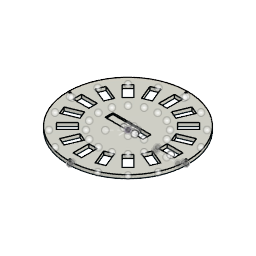
main (Autodesk Fusion 360 design; units mm, degrees)
Autodesk Fusion 360 part; units mm, degrees
sketch "Sketch1" plane through (0, 0, 0) normal (0, 0, 1) x (1, 0, 0)
  circle A0 centre (0, 0) radius 85
  line L0 (0, -85) -> (-7, -85) construction
  line L1 (0, -85) -> (7, -85) construction
  line L2 (-7, -85) -> (-7, -82) construction
  line L3 (7, -85) -> (7, -82) construction
  line L4 (7, -77) -> (5.9, -77) construction
  line L5 (7, -44.8) -> (5.9, -44.8) construction
  line L6 (-7, -44.8) -> (-5.9, -44.8) construction
  line L7 (-5.9, -44.8) -> (5.9, -44.8)
  line L8 (5.9, -44.8) -> (5.9, -77)
  line L9 (5.9, -77) -> (-5.9, -77)
  line L10 (-5.9, -77) -> (-5.9, -44.8)
  line L11 (0, -39.8) -> (0, -44.8) construction
  line L12 (11.6933, -43.6476) -> (22.5951, -39.132)
  line L13 (24.0157, -73.3966) -> (11.6933, -43.6476)
  line L14 (22.5951, -39.132) -> (34.9175, -68.8809)
  line L15 (34.9175, -68.8809) -> (24.0157, -73.3966)
  line L16 (27.5065, -35.8503) -> (35.8503, -27.5065)
  line L17 (50.2753, -58.6192) -> (27.5065, -35.8503)
  line L18 (35.8503, -27.5065) -> (58.6192, -50.2753)
  line L19 (58.6192, -50.2753) -> (50.2753, -58.6192)
  line L20 (39.132, -22.5951) -> (43.6476, -11.6933)
  line L21 (68.8809, -34.9175) -> (39.132, -22.5951)
  line L22 (43.6476, -11.6933) -> (73.3966, -24.0157)
  line L23 (73.3966, -24.0157) -> (68.8809, -34.9175)
  line L24 (44.8, -5.9) -> (44.8, 5.9)
  line L25 (77, -5.9) -> (44.8, -5.9)
  line L26 (44.8, 5.9) -> (77, 5.9)
  line L27 (77, 5.9) -> (77, -5.9)
  line L28 (43.6476, 11.6933) -> (39.132, 22.5951)
  line L29 (73.3966, 24.0157) -> (43.6476, 11.6933)
  line L30 (39.132, 22.5951) -> (68.8809, 34.9175)
  line L31 (68.8809, 34.9175) -> (73.3966, 24.0157)
  line L32 (35.8503, 27.5065) -> (27.5065, 35.8503)
  line L33 (58.6192, 50.2753) -> (35.8503, 27.5065)
  line L34 (27.5065, 35.8503) -> (50.2753, 58.6192)
  line L35 (50.2753, 58.6192) -> (58.6192, 50.2753)
  line L36 (22.5951, 39.132) -> (11.6933, 43.6476)
  line L37 (34.9175, 68.8809) -> (22.5951, 39.132)
  line L38 (11.6933, 43.6476) -> (24.0157, 73.3966)
  line L39 (24.0157, 73.3966) -> (34.9175, 68.8809)
  line L40 (5.9, 44.8) -> (-5.9, 44.8)
  line L41 (5.9, 77) -> (5.9, 44.8)
  line L42 (-5.9, 44.8) -> (-5.9, 77)
  line L43 (-5.9, 77) -> (5.9, 77)
  line L44 (-11.6933, 43.6476) -> (-22.5951, 39.132)
  line L45 (-24.0157, 73.3966) -> (-11.6933, 43.6476)
  line L46 (-22.5951, 39.132) -> (-34.9175, 68.8809)
  line L47 (-34.9175, 68.8809) -> (-24.0157, 73.3966)
  line L48 (-27.5065, 35.8503) -> (-35.8503, 27.5065)
  line L49 (-50.2753, 58.6192) -> (-27.5065, 35.8503)
  line L50 (-35.8503, 27.5065) -> (-58.6192, 50.2753)
  line L51 (-58.6192, 50.2753) -> (-50.2753, 58.6192)
  line L52 (-39.132, 22.5951) -> (-43.6476, 11.6933)
  line L53 (-68.8809, 34.9175) -> (-39.132, 22.5951)
  line L54 (-43.6476, 11.6933) -> (-73.3966, 24.0157)
  line L55 (-73.3966, 24.0157) -> (-68.8809, 34.9175)
  line L56 (-44.8, 5.9) -> (-44.8, -5.9)
  line L57 (-77, 5.9) -> (-44.8, 5.9)
  line L58 (-44.8, -5.9) -> (-77, -5.9)
  line L59 (-77, -5.9) -> (-77, 5.9)
  line L60 (-43.6476, -11.6933) -> (-39.132, -22.5951)
  line L61 (-73.3966, -24.0157) -> (-43.6476, -11.6933)
  line L62 (-39.132, -22.5951) -> (-68.8809, -34.9175)
  line L63 (-68.8809, -34.9175) -> (-73.3966, -24.0157)
  line L64 (-35.8503, -27.5065) -> (-27.5065, -35.8503)
  line L65 (-58.6192, -50.2753) -> (-35.8503, -27.5065)
  line L66 (-27.5065, -35.8503) -> (-50.2753, -58.6192)
  line L67 (-50.2753, -58.6192) -> (-58.6192, -50.2753)
  line L68 (-22.5951, -39.132) -> (-11.6933, -43.6476)
  line L69 (-34.9175, -68.8809) -> (-22.5951, -39.132)
  line L70 (-11.6933, -43.6476) -> (-24.0157, -73.3966)
  line L71 (-24.0157, -73.3966) -> (-34.9175, -68.8809)
  dimension "d1" = 170
  dimension "d2" = 7
  dimension "d3" = 7
  dimension "d4" = 3
  dimension "d5" = 3
  dimension "d7" = 5
  dimension "d8" = 1.1
  dimension "d10" = 1.1
  dimension "d11" = 1.1
  dimension "d15" = 360
  constraint coincident A0.centre origin
  constraint coincident A0 L0.start
  constraint horizontal L0
  constraint parallel L0 L1
  constraint perpendicular L0 L2
  constraint perpendicular L1 L3
  constraint perpendicular L7 L8
  constraint parallel L7 L9
  constraint parallel L8 L10
  constraint parallel L5 L7
  constraint midpoint L7 L11.end
  measures "d1" diameter of A0
  measures "d2" distance of L0.start L0.end
  measures "d3" distance of L0.start L1.end
  measures "d4" distance of L0.end L2.end
  measures "d5" distance of L1.end L3.end
  measures "d7" distance of L3.end L4.start
  measures "d8" distance of L4.start L4.end
  measures "d10" distance of L5.start L5.end
  measures "d11" distance of L6.start L6.end
extrude "Extrude1" add sketch "Sketch1" along normal blind 5
sketch "Sketch2" plane through (0, 0, 5) normal (0, 0, 1) x (-1, 0, 0)
  line L0 (-27.5065, -35.8503) -> (-50.2753, -58.6192)
  line L1 (-50.2753, -58.6192) -> (-58.6192, -50.2753)
  line L2 (-58.6192, -50.2753) -> (-35.8503, -27.5065)
  line L3 (-35.8503, -27.5065) -> (-27.5065, -35.8503)
  line L4 (5.9, -44.8) -> (5.9, -77)
  line L5 (5.9, -77) -> (-5.9, -77)
  line L6 (-5.9, -77) -> (-5.9, -44.8)
  line L7 (-5.9, -44.8) -> (5.9, -44.8)
  line L8 (-35.8503, 27.5065) -> (-58.6192, 50.2753)
  line L9 (-58.6192, 50.2753) -> (-50.2753, 58.6192)
  line L10 (-50.2753, 58.6192) -> (-27.5065, 35.8503)
  line L11 (-27.5065, 35.8503) -> (-35.8503, 27.5065)
  line L12 (35.8503, -27.5065) -> (58.6192, -50.2753)
  line L13 (58.6192, -50.2753) -> (50.2753, -58.6192)
  line L14 (50.2753, -58.6192) -> (27.5065, -35.8503)
  line L15 (27.5065, -35.8503) -> (35.8503, -27.5065)
  circle A0 centre (0, 0) radius 85
  line L16 (-5.9, 77) -> (5.9, 77)
  line L17 (5.9, 77) -> (5.9, 44.8)
  line L18 (5.9, 44.8) -> (-5.9, 44.8)
  line L19 (-5.9, 44.8) -> (-5.9, 77)
  line L20 (-39.132, -22.5951) -> (-68.8809, -34.9175)
  line L21 (-68.8809, -34.9175) -> (-73.3966, -24.0157)
  line L22 (-73.3966, -24.0157) -> (-43.6476, -11.6933)
  line L23 (-43.6476, -11.6933) -> (-39.132, -22.5951)
  line L24 (22.5951, -39.132) -> (34.9175, -68.8809)
  line L25 (34.9175, -68.8809) -> (24.0157, -73.3966)
  line L26 (24.0157, -73.3966) -> (11.6933, -43.6476)
  line L27 (11.6933, -43.6476) -> (22.5951, -39.132)
  line L28 (39.132, 22.5951) -> (68.8809, 34.9175)
  line L29 (68.8809, 34.9175) -> (73.3966, 24.0157)
  line L30 (73.3966, 24.0157) -> (43.6476, 11.6933)
  line L31 (43.6476, 11.6933) -> (39.132, 22.5951)
  line L32 (-22.5951, 39.132) -> (-34.9175, 68.8809)
  line L33 (-34.9175, 68.8809) -> (-24.0157, 73.3966)
  line L34 (-24.0157, 73.3966) -> (-11.6933, 43.6476)
  line L35 (-11.6933, 43.6476) -> (-22.5951, 39.132)
  line L36 (44.8, 5.9) -> (77, 5.9)
  line L37 (77, 5.9) -> (77, -5.9)
  line L38 (77, -5.9) -> (44.8, -5.9)
  line L39 (44.8, -5.9) -> (44.8, 5.9)
  line L40 (-11.6933, -43.6476) -> (-24.0157, -73.3966)
  line L41 (-24.0157, -73.3966) -> (-34.9175, -68.8809)
  line L42 (-34.9175, -68.8809) -> (-22.5951, -39.132)
  line L43 (-22.5951, -39.132) -> (-11.6933, -43.6476)
  line L44 (-43.6476, 11.6933) -> (-73.3966, 24.0157)
  line L45 (-73.3966, 24.0157) -> (-68.8809, 34.9175)
  line L46 (-68.8809, 34.9175) -> (-39.132, 22.5951)
  line L47 (-39.132, 22.5951) -> (-43.6476, 11.6933)
  line L48 (27.5065, 35.8503) -> (50.2753, 58.6192)
  line L49 (50.2753, 58.6192) -> (58.6192, 50.2753)
  line L50 (58.6192, 50.2753) -> (35.8503, 27.5065)
  line L51 (35.8503, 27.5065) -> (27.5065, 35.8503)
  line L52 (43.6476, -11.6933) -> (73.3966, -24.0157)
  line L53 (73.3966, -24.0157) -> (68.8809, -34.9175)
  line L54 (68.8809, -34.9175) -> (39.132, -22.5951)
  line L55 (39.132, -22.5951) -> (43.6476, -11.6933)
  line L56 (-44.8, -5.9) -> (-77, -5.9)
  line L57 (-77, -5.9) -> (-77, 5.9)
  line L58 (-77, 5.9) -> (-44.8, 5.9)
  line L59 (-44.8, 5.9) -> (-44.8, -5.9)
  line L60 (11.6933, 43.6476) -> (24.0157, 73.3966)
  line L61 (24.0157, 73.3966) -> (34.9175, 68.8809)
  line L62 (34.9175, 68.8809) -> (22.5951, 39.132)
  line L63 (22.5951, 39.132) -> (11.6933, 43.6476)
  line L64 (0, 0) -> (0, 5.5) construction
  line L65 (0, 5.5) -> (27, 5.5) construction
  line L66 (27, 5.5) -> (27, -5.5) construction
  line L67 (27, -5.5) -> (-27, -5.5) construction
  line L68 (27, 5.5) -> (27, -5.5)
  line L69 (27, -5.5) -> (-27, -5.5)
  line L70 (-27, -5.5) -> (-27, 5.5)
  line L71 (-27, 5.5) -> (27, 5.5)
  dimension "d22" = 5.5
  dimension "d23" = 27
  dimension "d24" = 11
  dimension "d25" = 54
  constraint coincident A0.centre L64.start
  constraint vertical L64
  constraint perpendicular L64 L65
  constraint perpendicular L65 L66
  constraint perpendicular L66 L67
  constraint perpendicular L68 L69
  constraint parallel L68 L70
  constraint parallel L69 L71
  measures "d22" distance of A0.centre L64.end
  measures "d23" distance of L64.end L65.end
  measures "d24" distance of L65.end L66.end
  measures "d25" distance of L66.end L67.end
extrude "Extrude2" cut sketch "Sketch2" against normal blind 2 contours L68 L69 L70 L71
sketch "Sketch3" plane through (0, 0, 3) normal (0, 0, 1) x (-1, 0, 0)
  line L0 (-27, 5.5) -> (-27, -5.5)
  line L1 (-27, -5.5) -> (27, -5.5)
  line L2 (27, -5.5) -> (27, 5.5)
  line L3 (27, 5.5) -> (-27, 5.5)
  line L4 (-27, -5.5) -> (-12.1144, -5.5)
  line L5 (-12.1144, -5.5) -> (-12.1144, 5.5)
  line L6 (-12.1144, 5.5) -> (-27, 5.5)
  line L7 (-27, 5.5) -> (-27, -5.5)
  constraint horizontal L4
  constraint vertical L5
  constraint horizontal L6
  constraint vertical L7
  constraint coincident L3 L5.end
  constraint coincident L0.end L1.start
extrude "Extrude3" cut sketch "Sketch3" against normal blind 39 contours L0 L1 L3 L4 L5 L6 L7
sketch "Sketch4" plane through (0, 0, 0) normal (0, 0, -1) x (1, 0, 0)
  line L0 (-24.0157, 73.3966) -> (-11.6933, 43.6476)
  line L1 (-11.6933, 43.6476) -> (-22.5951, 39.132)
  line L2 (-22.5951, 39.132) -> (-34.9175, 68.8809)
  line L3 (-34.9175, 68.8809) -> (-24.0157, 73.3966)
  line L4 (77, -5.9) -> (44.8, -5.9)
  line L5 (44.8, -5.9) -> (44.8, 5.9)
  line L6 (44.8, 5.9) -> (77, 5.9)
  line L7 (77, 5.9) -> (77, -5.9)
  line L8 (-73.3966, -24.0157) -> (-43.6476, -11.6933)
  line L9 (-43.6476, -11.6933) -> (-39.132, -22.5951)
  line L10 (-39.132, -22.5951) -> (-68.8809, -34.9175)
  line L11 (-68.8809, -34.9175) -> (-73.3966, -24.0157)
  line L12 (-50.2753, 58.6192) -> (-27.5065, 35.8503)
  line L13 (-27.5065, 35.8503) -> (-35.8503, 27.5065)
  line L14 (-35.8503, 27.5065) -> (-58.6192, 50.2753)
  line L15 (-58.6192, 50.2753) -> (-50.2753, 58.6192)
  line L16 (73.3966, 24.0157) -> (43.6476, 11.6933)
  line L17 (43.6476, 11.6933) -> (39.132, 22.5951)
  line L18 (39.132, 22.5951) -> (68.8809, 34.9175)
  line L19 (68.8809, 34.9175) -> (73.3966, 24.0157)
  line L20 (24.0157, -73.3966) -> (11.6933, -43.6476)
  line L21 (11.6933, -43.6476) -> (22.5951, -39.132)
  line L22 (22.5951, -39.132) -> (34.9175, -68.8809)
  line L23 (34.9175, -68.8809) -> (24.0157, -73.3966)
  line L24 (-77, 5.9) -> (-44.8, 5.9)
  line L25 (-44.8, 5.9) -> (-44.8, -5.9)
  line L26 (-44.8, -5.9) -> (-77, -5.9)
  line L27 (-77, -5.9) -> (-77, 5.9)
  line L28 (34.9175, 68.8809) -> (22.5951, 39.132)
  line L29 (22.5951, 39.132) -> (11.6933, 43.6476)
  line L30 (11.6933, 43.6476) -> (24.0157, 73.3966)
  line L31 (24.0157, 73.3966) -> (34.9175, 68.8809)
  line L32 (-68.8809, 34.9175) -> (-39.132, 22.5951)
  line L33 (-39.132, 22.5951) -> (-43.6476, 11.6933)
  line L34 (-43.6476, 11.6933) -> (-73.3966, 24.0157)
  line L35 (-73.3966, 24.0157) -> (-68.8809, 34.9175)
  line L36 (-34.9175, -68.8809) -> (-22.5951, -39.132)
  line L37 (-22.5951, -39.132) -> (-11.6933, -43.6476)
  line L38 (-11.6933, -43.6476) -> (-24.0157, -73.3966)
  line L39 (-24.0157, -73.3966) -> (-34.9175, -68.8809)
  line L40 (68.8809, -34.9175) -> (39.132, -22.5951)
  line L41 (39.132, -22.5951) -> (43.6476, -11.6933)
  line L42 (43.6476, -11.6933) -> (73.3966, -24.0157)
  line L43 (73.3966, -24.0157) -> (68.8809, -34.9175)
  line L44 (-5.9, 77) -> (5.9, 77)
  line L45 (5.9, 77) -> (5.9, 44.8)
  line L46 (5.9, 44.8) -> (-5.9, 44.8)
  line L47 (-5.9, 44.8) -> (-5.9, 77)
  circle A0 centre (0, 0) radius 85
  line L48 (-58.6192, -50.2753) -> (-35.8503, -27.5065)
  line L49 (-35.8503, -27.5065) -> (-27.5065, -35.8503)
  line L50 (-27.5065, -35.8503) -> (-50.2753, -58.6192)
  line L51 (-50.2753, -58.6192) -> (-58.6192, -50.2753)
  line L52 (58.6192, 50.2753) -> (35.8503, 27.5065)
  line L53 (35.8503, 27.5065) -> (27.5065, 35.8503)
  line L54 (27.5065, 35.8503) -> (50.2753, 58.6192)
  line L55 (50.2753, 58.6192) -> (58.6192, 50.2753)
  line L56 (-5.9, -77) -> (-5.9, -44.8)
  line L57 (-5.9, -44.8) -> (5.9, -44.8)
  line L58 (5.9, -44.8) -> (5.9, -77)
  line L59 (5.9, -77) -> (-5.9, -77)
  line L60 (50.2753, -58.6192) -> (27.5065, -35.8503)
  line L61 (27.5065, -35.8503) -> (35.8503, -27.5065)
  line L62 (35.8503, -27.5065) -> (58.6192, -50.2753)
  line L63 (58.6192, -50.2753) -> (50.2753, -58.6192)
  line L64 (27, -5.5) -> (12.1144, -5.5)
  line L65 (12.1144, -5.5) -> (12.1144, 5.5)
  line L66 (12.1144, 5.5) -> (27, 5.5)
  line L67 (27, 5.5) -> (27, -5.5)
  line L68 (44.8, 0) -> (42.3, 0) construction
  line L69 (44.8, 5.9) -> (77, 5.9) construction
  line L70 (60.9, 5.9) -> (60.9, 0.1412) construction
  circle A1 centre (42.3, 0) radius 0.75
  circle A2 centre (79.5, 0) radius 0.75
  line L71 (60.9, 5.9) -> (60.9, 0.1412) construction
  circle A3 centre (73.4484, 30.4233) radius 0.75
  circle A4 centre (39.0801, 16.1875) radius 0.75
  circle A5 centre (56.215, 56.215) radius 0.75
  circle A6 centre (29.9106, 29.9106) radius 0.75
  circle A7 centre (30.4233, 73.4484) radius 0.75
  circle A8 centre (16.1875, 39.0801) radius 0.75
  circle A9 centre (0, 79.5) radius 0.75
  circle A10 centre (0, 42.3) radius 0.75
  circle A11 centre (-30.4233, 73.4484) radius 0.75
  circle A12 centre (-16.1875, 39.0801) radius 0.75
  circle A13 centre (-56.215, 56.215) radius 0.75
  circle A14 centre (-29.9106, 29.9106) radius 0.75
  circle A15 centre (-73.4484, 30.4233) radius 0.75
  circle A16 centre (-39.0801, 16.1875) radius 0.75
  circle A17 centre (-79.5, 0) radius 0.75
  circle A18 centre (-42.3, 0) radius 0.75
  circle A19 centre (-73.4484, -30.4233) radius 0.75
  circle A20 centre (-39.0801, -16.1875) radius 0.75
  circle A21 centre (-56.215, -56.215) radius 0.75
  circle A22 centre (-29.9106, -29.9106) radius 0.75
  circle A23 centre (-30.4233, -73.4484) radius 0.75
  circle A24 centre (-16.1875, -39.0801) radius 0.75
  circle A25 centre (0, -79.5) radius 0.75
  circle A26 centre (0, -42.3) radius 0.75
  circle A27 centre (30.4233, -73.4484) radius 0.75
  circle A28 centre (16.1875, -39.0801) radius 0.75
  circle A29 centre (56.215, -56.215) radius 0.75
  circle A30 centre (29.9106, -29.9106) radius 0.75
  circle A31 centre (73.4484, -30.4233) radius 0.75
  circle A32 centre (39.0801, -16.1875) radius 0.75
  line L72 (0, 79.5) -> (0, 82.5) construction
  circle A33 centre (0, 82.5) radius 1.55
  line L73 (0, 0) -> (0, 12.2218) construction
  line L74 (0, 12.2218) -> (0, 0) construction
  line L75 (0, 0) -> (-5.8676, 0) construction
  line L76 (0, 0) -> (6.7946, 0) construction
  circle A34 centre (0, -82.5) radius 1.55
  line L77 (79.5, 0) -> (82.5, 0) construction
  circle A35 centre (82.5, 0) radius 1.55
  line L78 (0, 0) -> (0, -8.2494) construction
  circle A36 centre (-82.5, 0) radius 1.55
  line L79 (0, 0) -> (-15.877, 16.4411) construction
  line L80 (0, 0) -> (22.8559, 0) construction
  line L81 (0, 0) -> (7.0711, -7.0711) construction
  line L82 (0, 0) -> (10, 0) construction
  line L83 (0, 0) -> (7.0711, 7.0711) construction
  line L84 (0, 0) -> (10, 0) construction
  line L85 (0, 0) -> (-6.6532, -6.6532) construction
  line L86 (0, 0) -> (9.4097, 0) construction
  dimension "d30" = 2.5
  dimension "d31" = 1.5
  dimension "d33" = 360
  dimension "d36" = 3
  dimension "d37" = 3.1
  dimension "d38" = 3
  dimension "d39" = 3.1
  dimension "d40" = 134
  dimension "d41" = 45
  dimension "d42" = 10
  dimension "d43" = 10
  dimension "d44" = 45
  dimension "d45" = 135
  constraint midpoint L5 L68.start
  constraint perpendicular L5 L68
  constraint coincident L5.end L6.start
  constraint coincident L6.end L7.start
  constraint midpoint L69 L70.start
  constraint perpendicular L6 L70
  constraint coincident L68.end A1.centre
  constraint symmetric L71.start L70 L70.start
  constraint symmetric L71.end L70 L70.end
  constraint symmetric L70 A1 A2
  constraint coincident A9.centre L72.start
  constraint vertical L72
  constraint coincident L72.end A33.centre
  constraint coincident A0.centre L73.start
  constraint perpendicular L66 L73
  constraint perpendicular L74 L75
  constraint perpendicular L73 L76
  constraint symmetric A33 L75 A34
  constraint coincident A2.centre L77.start
  constraint perpendicular L7 L77
  constraint coincident L77.end A35.centre
  constraint perpendicular L76 L78
  constraint symmetric A35 L78 A36
  constraint horizontal L80
  constraint horizontal L82
  constraint horizontal L84
  constraint horizontal L86
  measures "d30" distance of L68.start L68.end
  measures "d31" diameter of A1
  measures "d36" distance of A9.centre L72.end
  measures "d37" diameter of A33
  measures "d38" distance of A2.centre L77.end
  measures "d39" diameter of A35
  measures "d40" angle of L79 L80
  measures "d41" angle of L81 L82
  measures "d42" distance of A0.centre L81.end
  measures "d43" distance of A0.centre L83.end
  measures "d44" angle of L83 L84
  measures "d45" angle of L85 L86
extrude "Extrude4" cut sketch "Sketch4" against normal blind 3.5 contours A1 | A2 | A3 | A4 | A5 | A6 | A7 | A8 | A9 | A10 | A11 | A12 | A13 | A14 | A15 | A16 | A17 | A18 | A19 | A20 | A21 | A22 | A23 | A24 | A25 | A26 | A27 | A28 | A29 | A30 | A31 | A32
extrude "Extrude5" cut sketch "Sketch4" against normal blind 5 contours A33 | A34 | A35 | A36
thread "Thread1" "ISO Metric profile 3.0 M3x0.5 M3x0.5 6H" major diameter 3.086 minor diameter 2.529 pitch 0.5 angle 60 resizes the face on face at (-83.5823, -1.1096, 3.3333)
thread "Thread2" "ISO Metric profile 3.0 M3x0.5 M3x0.5 6H" major diameter 3.086 minor diameter 2.529 pitch 0.5 angle 60 resizes the face on face at (1.5481, -82.4227, 3.3333)
thread "Thread3" "ISO Metric profile 3.0 M3x0.5 M3x0.5 6H" major diameter 3.086 minor diameter 2.529 pitch 0.5 angle 60 resizes the face on face at (81.4177, -1.1096, 3.3333)
thread "Thread4" "ISO Metric profile 3.0 M3x0.5 M3x0.5 6H" major diameter 3.086 minor diameter 2.529 pitch 0.5 angle 60 resizes the face on face at (1.5481, 82.5773, 3.3333)
extrude "Extrude6" add 1 faces at (1.9667, -77, 1.6667) along direction (0, 1, 0) blind 5
extrude "Extrude7" add 1 faces at (-27.6497, -71.8913, 1.6667) along direction (0.382683, 0.92388, 0) blind 5
extrude "Extrude8" add 1 faces at (-53.0566, -55.8379, 1.6667) along direction (0.707107, 0.707107, 0) blind 5
extrude "Extrude9" add 1 faces at (-70.3861, -31.2836, 1.6667) along direction (0.92388, 0.382683, 0) blind 5
extrude "Extrude10" add 1 faces at (31.2836, -70.3861, 1.6667) along direction (-0.382683, 0.92388, 0) blind 5
extrude "Extrude11" add 1 faces at (55.8379, -53.0566, 1.6667) along direction (-0.707107, 0.707107, 0) blind 5
extrude "Extrude12" add 1 faces at (71.8913, -27.6497, 1.6667) along direction (-0.92388, 0.382683, 0) blind 5
extrude "Extrude13" add 1 faces at (77, 1.9667, 1.6667) along direction (-1, 0, 0) blind 5
extrude "Extrude14" add 1 faces at (70.3861, 31.2836, 1.6667) along direction (-0.92388, -0.382683, 0) blind 5
extrude "Extrude15" add 1 faces at (53.0566, 55.8379, 1.6667) along direction (-0.707107, -0.707107, 0) blind 5
extrude "Extrude16" add 1 faces at (27.6497, 71.8913, 1.6667) along direction (-0.382683, -0.92388, 0) blind 5
extrude "Extrude17" add 1 faces at (-1.9667, 77, 3.3333) along direction (0, -1, 0) blind 5
extrude "Extrude18" add 1 faces at (-31.2836, 70.3861, 1.6667) along direction (0.382683, -0.92388, 0) blind 5
extrude "Extrude19" add 1 faces at (-55.8379, 53.0566, 3.3333) along direction (0.707107, -0.707107, 0) blind 5
extrude "Extrude20" add 1 faces at (-71.8913, 27.6497, 1.6667) along direction (0.92388, -0.382683, 0) blind 5
extrude "Extrude21" add 1 faces at (-77, -1.9667, 1.6667) along direction (1, 0, 0) blind 5
extrude "Extrude22" add 1 faces at (-44.8, 1.9667, 1.6667) along direction (-1, 0, 0) blind 5
extrude "Extrude23" add 1 faces at (-42.1424, -15.3273, 1.6667) along direction (-0.92388, -0.382683, 0) blind 5
extrude "Extrude24" add 1 faces at (-33.069, -30.2877, 1.6667) along direction (-0.707107, -0.707107, 0) blind 5
extrude "Extrude25" add 1 faces at (-18.9612, -40.6372, 1.6667) along direction (-0.382683, -0.92388, 0) blind 5
extrude "Extrude26" add 1 faces at (-1.9667, -44.8, 1.6667) along direction (0, -1, 0) blind 5
extrude "Extrude27" add 1 faces at (15.3273, -42.1424, 1.6667) along direction (0.382683, -0.92388, 0) blind 5
extrude "Extrude28" add 1 faces at (30.2877, -33.069, 1.6667) along direction (0.707107, -0.707107, 0) blind 5
extrude "Extrude29" add 1 faces at (40.6372, -18.9612, 1.6667) along direction (0.92388, -0.382683, 0) blind 5
extrude "Extrude30" add 1 faces at (44.8, -1.9667, 1.6667) along direction (1, 0, 0) blind 5
extrude "Extrude31" add 1 faces at (42.1424, 15.3273, 1.6667) along direction (0.92388, 0.382683, 0) blind 5
extrude "Extrude32" add 1 faces at (33.069, 30.2877, 1.6667) along direction (0.707107, 0.707107, 0) blind 5
extrude "Extrude33" add 1 faces at (15.3273, 42.1424, 3.3333) along direction (0.382683, 0.92388, 0) blind 5
extrude "Extrude34" add 1 faces at (1.9667, 44.8, 1.6667) along direction (0, 1, 0) blind 5
extrude "Extrude35" add 1 faces at (-15.3273, 42.1424, 3.3333) along direction (-0.382683, 0.92388, 0) blind 5
extrude "Extrude36" add 1 faces at (-33.069, 30.2877, 1.6667) along direction (-0.707107, 0.707107, 0) blind 5
extrude "Extrude37" add 1 faces at (-40.6372, 18.9612, 1.6667) along direction (-0.92388, 0.382683, 0) blind 5
